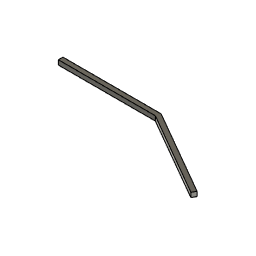
angle (Autodesk Fusion 360 design; units mm, degrees)
Autodesk Fusion 360 part; units mm, degrees
sketch "Sketch1" plane through (0, 0, 0) normal (0, 0, 1) x (1, 0, 0)
  line L0 (0.5, 3.925) -> (8.0469, 3.925)
  line L1 (7.9531, 3.575) -> (0.5, 3.575)
  line L2 (0.5, 3.575) -> (0.5, 3.925)
  line L3 (0.5, 3.75) -> (8, 3.75) construction
  line L4 (8, 3.75) -> (14.4952, 0) construction
  line L5 (8.0469, 3.925) -> (14.5827, 0.1516)
  line L6 (14.5827, 0.1516) -> (14.4077, -0.1516)
  line L7 (14.4077, -0.1516) -> (7.9531, 3.575)
  dimension "d1" = 150
  dimension "d2" = 0.35
  dimension "d3" = 0.35
  dimension "d14" = 7.5
  dimension "d15" = 7.5
  dimension "d16" = 3.75
  dimension "d20" = 0.5
  constraint horizontal L0
  constraint horizontal L1
  constraint vertical L2
  constraint midpoint L2 L3.start
  constraint midpoint L4.end L6
  constraint parallel L4 L5
  constraint parallel L5 L7
  constraint coincident L0.end L5.start
  constraint horizontal L3
  constraint perpendicular L6 L7
  constraint coincident L3.end L4.start
  measures "d1" angle of L3 L4
  measures "d2" distance of L0 L1
  measures "d3" distance of L5 L7
  measures "d14" distance of L3.end L4.end
  measures "d15" distance of L3.start L3.end
  measures "d16" vertical distance of origin L3.start
  measures "d20" horizontal distance of origin L3.start
extrude "Extrude1" add sketch "Sketch1" along normal blind 0.35
equation "d1 = angle"
equation "d2 = channelwidth"
equation "d3 = d2"
equation "angle = 150 deg"
equation "channelwidth = 0.35 mm"
equation "length = 7.5 mm"
equation "length2 = 7.5 mm"
equation "depth = 0.35 mm"
equation "d11 = depth"
equation "d14 = length2"
equation "d15 = length"
equation "d16 = yoffset"
equation "yoffset = length2 * cos(angle - 90 deg)"
equation "xoffset = 0.5 mm"
equation "d20 = xoffset"
